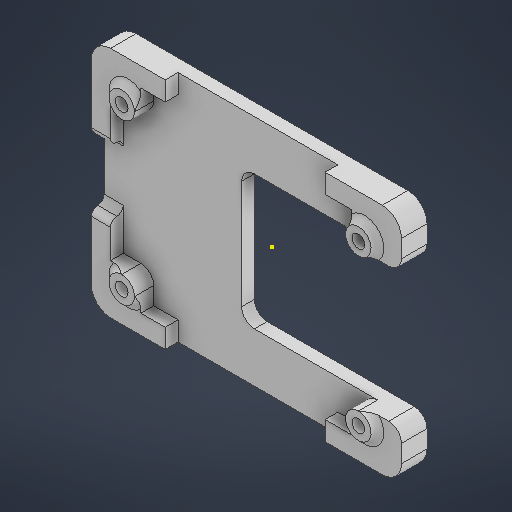
# Autodesk Inventor part: 陀螺仪外壳
Saved by Autodesk Inventor 2025 (Build 290162000, 162)
## iProperties
Created: 2025-01-04
Part Number: 陀螺仪外壳
Material: 常规
Document SubType Name: Modeling
Designer: HZD
Density: 1 g/cm^3
Appearance: 默认
Author: HZD
Autodesk Inventor part; units mm, degrees
ref_plane "YZ Plane" through (0, 0, 0) normal (1, 0, 0) x (0, 1, 0)
ref_plane "XZ Plane" through (0, 0, 0) normal (0, 1, 0) x (-1, 0, 0)
ref_plane "XY Plane" through (0, 0, 0) normal (0, 0, 1) x (1, 0, 0)
sketch "草图1" plane through (0, 0, 0) normal (0, 0, 1) x (1, 0, 0)
  line L0 (21.25, -15.25) -> (-21.25, -15.25)
  line L1 (-21.25, -15.25) -> (-21.25, 15.25)
  line L2 (-21.25, 15.25) -> (21.25, 15.25)
  line L3 (21.25, 15.25) -> (21.25, -15.25)
  line L4 (21.25, -15.25) -> (-21.25, 15.25) construction
  line L5 (-21.25, -15.25) -> (21.25, 15.25) construction
  line L6 (24.25, -18.25) -> (-24.25, -18.25)
  line L7 (-24.25, -18.25) -> (-24.25, 18.25)
  line L8 (-24.25, 18.25) -> (24.25, 18.25)
  line L9 (24.25, 18.25) -> (24.25, -18.25)
  point P0 (0, 0)
  dimension "d0" = 42.5
  dimension "d1" = 30.5
  dimension "d2" = 3
  constraints: 20 end point, 4 parallel, 2 midpoint, 2 perpendicular, 1 horizontal, 3 other
  measures "d0" distance of L1.end L2.end
  measures "d1" distance of L0.end L1.end
  measures "d2" distance between parallel lines of L3 L9
extrude "拉伸1" add sketch "草图1" along normal blind 2 contours L0 L1 L2 L3 | L6 L7 L8 L9
extrude "拉伸2" add sketch "草图1" along normal blind 4
fillet "圆角1" radius 3 4 edges at (24.25, 18.25, 2) (-24.25, 18.25, 2) (-24.25, -18.25, 2) (24.25, -18.25, 2)
sketch "草图2" plane through (0, 0, 2) normal (0, 0, 1) x (1, 0, 0)
  circle A0 centre (-18.5, 12.5) radius 1
  line L0 (21.25, 18.25) -> (-21.25, 18.25) projected
  line L1 (0, 18.25) -> (0, 0)
  line L2 (-24.25, 15.25) -> (-24.25, -15.25) projected
  line L3 (-24.25, 0) -> (0, 0)
  circle A1 centre (-18.5, 12.5) radius 2
  line L4 (-16.5, 12.5) -> (-16.5, 15.8598)
  line L5 (-16.5, 15.8598) -> (-22.5422, 15.8598)
  line L6 (-22.5422, 15.8598) -> (-22.5422, 10.5)
  line L7 (-22.5422, 10.5) -> (-18.5, 10.5)
  dimension "d8" = 2
  dimension "d9" = 18.5
  dimension "d10" = 12.5
  dimension "d11" = 4
  constraints: 12 end point, 3 perpendicular, 2 centre point, 2 midpoint, 2 point on circle, 2 vertical, 1 coincident, 1 tangent
  measures "d8" diameter of A0
  measures "d9" distance from line of A0.centre L1
  measures "d10" distance from line of L3 A0.centre
  measures "d11" diameter of A1
extrude "拉伸3" add sketch "草图2" along normal blind 2
extrude "拉伸4" cut sketch "草图2" against normal blind 4 contours A0
mirror "镜像1" about plane through (0, 0, 0) normal (1, 0, 0) of "拉伸4", "拉伸3"
mirror "镜像2" about plane through (0, 0, 0) normal (0, 1, 0) of "拉伸3", "拉伸4", "镜像1"
sketch "草图3" plane through (0, 0, 0) normal (-1, 0, 0) x (0, -1, 0)
  point P0 (0, 0)
sketch "草图5" plane through (0, 0, 2) normal (0, 0, 1) x (1, 0, 0)
  line L0 (-2.75, -10.5) -> (24.25, -10.5)
  line L1 (24.25, -10.5) -> (24.25, 10.5)
  line L2 (24.25, 10.5) -> (-2.75, 10.5)
  line L3 (-2.75, 10.5) -> (-2.75, -10.5)
  line L4 (-2.75, -10.5) -> (24.25, 10.5) construction
  line L5 (24.25, -10.5) -> (-2.75, 10.5) construction
  line L6 (24.25, -15.25) -> (24.25, 15.25) projected
  point P0 (0, 0)
  point P1 (10.75, 0)
  dimension "d21" = 21
  dimension "d22" = 27
  constraints: 12 end point, 2 midpoint, 2 parallel, 1 collinear, 1 horizontal, 1 perpendicular
  measures "d21" distance of L0.end L1.end
  measures "d22" distance between parallel lines of L1 L3
extrude "拉伸6" cut sketch "草图5" along normal mid plane 19.25
fillet "圆角3" radius 2 4 edges at (24.25, 10.5, 2) (24.25, -10.5, 2) (-2.75, -10.5, 1) (-2.75, 10.5, 1)
sketch "草图6" plane through (0, 0, 4) normal (0, 0, 1) x (1, 0, 0)
  line L0 (-18.8511, 5) -> (-26.9848, 5)
  line L1 (-26.9848, 5) -> (-26.9848, -5)
  line L2 (-26.9848, -5) -> (-18.8511, -5)
  line L3 (-18.8511, -5) -> (-18.8511, 5)
  line L4 (-18.8511, 5) -> (-26.9848, -5) construction
  line L5 (-26.9848, 5) -> (-18.8511, -5) construction
  point P0 (0, 0)
  point P1 (-22.9179, 0)
  point P2 (-22.9179, -5)
  point P3 (-22.9179, 5)
  dimension "d26" = 10
  constraints: 12 end point, 4 midpoint, 2 parallel, 1 horizontal, 1 perpendicular
  measures "d26" distance of point (-22.918, -5) point (-22.918, 5)
extrude "拉伸7" cut sketch "草图6" against normal up to surface (2 mm away)
fillet "圆角4" radius 1 4 edges at (-22.75, -5, 4) (-22.75, 5, 4) (-22.75, 5, 2) (-22.75, -5, 2)
sketch "草图7" plane through (0, 0, 4) normal (0, 0, 1) x (1, 0, 0)
  circle A0 centre (-18.5, 12.5) radius 1 projected
  circle A1 centre (18.5, 12.5) radius 1 projected
  circle A2 centre (18.5, -12.5) radius 1 projected
  circle A3 centre (-18.5, -12.5) radius 1 projected
  circle A4 centre (-18.5, -12.5) radius 2
  circle A5 centre (-18.5, 12.5) radius 2
  circle A6 centre (18.5, 12.5) radius 2
  circle A7 centre (18.5, -12.5) radius 2
  point P0 (0, 0)
  constraints: 4 centre point, 4 coincident
extrude "拉伸8" add sketch "草图7" along normal blind 1
fillet "圆角5" radius 1 6 edges at (-19.9142, 13.9142, 4) (19.9142, 11.0858, 4) (18.5, 14.5, 4) (18.5, -14.5, 4) (19.9142, -11.0858, 4) (-19.9142, -13.9142, 4)
sketch "草图8" plane through (-21.25, -18.25, 0) normal (0, -1, 0) x (1, 0, 0)
  line L0 (-0.0206, 5.6521) -> (42.4794, 5.6521)
  line L1 (37.75, 2) -> (4.75, 2) projected
  line L2 (8.5519, 5.6521) -> (33.5519, 5.6521)
  line L3 (33.5519, 5.6521) -> (33.5519, 2)
  line L4 (33.5519, 2) -> (8.5519, 2)
  line L5 (8.5519, 2) -> (8.5519, 5.6521)
  point P0 (21.25, 0)
  point P1 (8.5519, 3.826)
  point P2 (33.5519, 3.826)
  dimension "d33" = 25
  constraints: 10 end point, 2 midpoint, 2 parallel, 2 point on line, 1 horizontal, 1 perpendicular
  measures "d33" distance of point (8.552, 3.826) point (33.552, 3.826)
extrude "拉伸9" cut sketch "草图8" against normal blind 39.25
ref_plane "工作平面1" through (0, 0, 0) normal (1, 0, 0) x (0, 1, 0)
ref_plane "工作平面2" through (0, 0, 0) normal (-1, 0, 0) x (0, -1, 0)
ref_plane "工作平面3" through (0, 0, 0) normal (-1, 0, 0) x (0, -1, 0)
equation "\"d14\" = d11"
